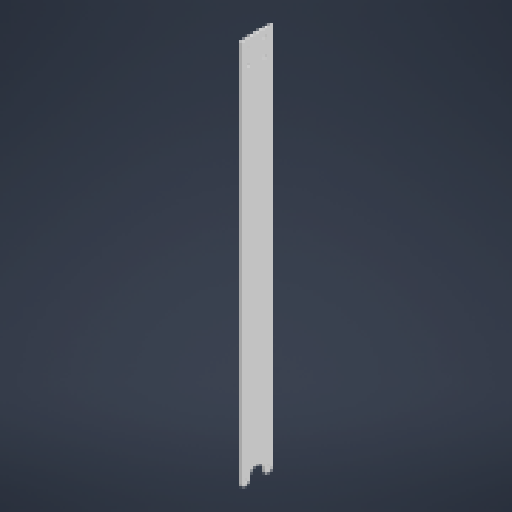
# Autodesk Inventor part: DropBar
Saved by Autodesk Inventor 2024.1 (Build 281209000, 209)
## iProperties
Created: 2023-10-25
Part Number: DropBar
Material: Generic
Document SubType Name: Modeling
Designer: Brandon
Density: 1 g/cm^3
Appearance: Default
Author: Brandon
Autodesk Inventor part; units mm, degrees
ref_plane "YZ Plane" through (0, 0, 0) normal (1, 0, 0) x (0, 1, 0)
ref_plane "XZ Plane" through (0, 0, 0) normal (0, 1, 0) x (-1, 0, 0)
ref_plane "XY Plane" through (0, 0, 0) normal (0, 0, 1) x (1, 0, 0)
sketch "Sketch1" plane through (0, 0, 0) normal (1, 0, 0) x (0, 1, 0)
  line L0 (0, 0) -> (609.6, 0)
  line L1 (609.6, 0) -> (609.6, -50.8)
  line L2 (609.6, -50.8) -> (0, -50.8)
  line L3 (0, -50.8) -> (0, 0)
  circle A0 centre (8.89, -25.4) radius 11.049
  circle A1 centre (8.89, -7.62) radius 2
  circle A2 centre (8.89, -43.18) radius 2
  circle A3 centre (596.9, -12.7) radius 2
  circle A4 centre (596.9, -38.1) radius 2
  circle A5 centre (571.5, -12.7) radius 2
  circle A6 centre (571.5, -38.1) radius 2
  point P0 (0, -25.4)
  point P1 (0, -18.8389)
  point P2 (0, -31.9611)
  dimension "d0" = 609.6
  dimension "d1" = 50.8
  dimension "d2" = 22.098
  dimension "d3" = 8.89
  dimension "d4" = 4
  dimension "d5" = 4
  dimension "d6" = 7.62
  dimension "d7" = 8.89
  dimension "d8" = 7.62
  dimension "d9" = 8.89
  dimension "d10" = 4
  dimension "d11" = 4
  dimension "d12" = 4
  dimension "d13" = 4
  dimension "d14" = 25.4
  dimension "d15" = 25.4
  dimension "d16" = 25.4
  dimension "d17" = 25.4
  dimension "d18" = 12.7
  dimension "d19" = 12.7
  constraints: 8 end point, 7 centre point, 2 horizontal alignment, 2 parallel, 1 horizontal, 1 midpoint, 1 perpendicular, 1 vertical alignment
  measures "d0" distance of L1.end L2.end
  measures "d1" distance of L0.end L1.end
  measures "d2" diameter of A0
  measures "d3" distance of point (0, -25.4) A0.centre
  measures "d4" diameter of A1
  measures "d5" diameter of A2
  measures "d6" distance from line of L0 A1.centre
  measures "d7" distance from line of L3 A1.centre
  measures "d8" distance from line of L2 A2.centre
  measures "d9" distance from line of L3 A2.centre
  measures "d10" diameter of A3
  measures "d11" diameter of A4
  measures "d12" diameter of A5
  measures "d13" diameter of A6
  measures "d14" distance of A5.centre A3.centre
  measures "d15" distance of A4.centre A3.centre
  measures "d16" distance of A6.centre A4.centre
  measures "d17" distance of A6.centre A5.centre
  measures "d18" distance from line of L0 A3.centre
  measures "d19" distance from line of L1 A3.centre
extrude "Extrusion1" add sketch "Sketch1" along normal blind 3 contours L0 L1 L2 L3 A0
fillet "Fillet1" radius 6.35 4 edges at (1.5, 0, -31.9611) (1.5, 0, -18.8389) (1.5, 0, 0) (1.5, 0, -50.8)
body "Solid1"
